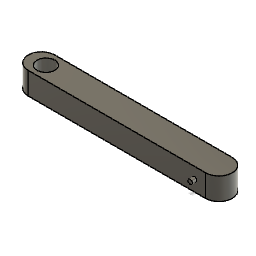
Segunda parte Braço v7 (Autodesk Fusion 360 design; units mm, degrees)
Autodesk Fusion 360 part; units mm, degrees
note: some values were not read from the file. Set by a fixed rule: which sketch regions a step uses.
sketch "Sketch1" plane through (0, 0, 0) normal (0, 1, 0) x (1, 0, 0)
  line L0 (100, -15) -> (-100, -15)
  line L1 (-100, -15) -> (-100, 15)
  line L2 (-100, 15) -> (100, 15)
  line L3 (100, 15) -> (100, -15)
  line L4 (100, -15) -> (-100, 15) construction
  line L5 (-100, -15) -> (100, 15) construction
  arc A0 (-95.599, 14.3399) -> (-95.599, -14.3399) centre (-100, 0) ccw
  arc A1 (95.599, -14.3399) -> (95.599, 14.3399) centre (100, 0) ccw
  dimension "d1" = 200
  dimension "d2" = 30
  constraint horizontal L0
  constraint perpendicular L0 L1
  constraint parallel L0 L2
  constraint parallel L1 L3
  constraint coincident L4 origin
  constraint coincident L5 origin
  constraint midpoint L3 A1.centre
  constraint coincident L2.end A1
  constraint midpoint L1 A0.centre
  constraint coincident L1.end A0
  constraint coincident L5 A0.end
  constraint coincident L4 A0.start
  constraint coincident L5 A1.end
  constraint coincident L4 A1.start
  measures "d1" distance of L1.end L2.end
  measures "d2" distance of L0.end L1.end
extrude "Extrude1" add sketch "Sketch1" along normal blind 25 makes body 1
sketch "Sketch2" plane through (0, 25, 0) normal (0, 1, 0) x (-1, 0, 0)
  arc A0 (100, -15) -> (100, 15) centre (100, 0) ccw
  line L0 (100, 15) -> (-100, 15)
  arc A1 (-100, 15) -> (-100, -15) centre (-100, 0) ccw
  line L1 (-100, -15) -> (100, -15)
  circle A2 centre (95, 0) radius 10
  dimension "d6" = 20
  measures "d6" diameter of A2
extrude "Extrude2" cut sketch "Sketch2" against normal blind 70 contours A2 bodies 1
sketch "Sketch3" plane through (0, 0, -15) normal (0, 0, -1) x (-1, 0, 0)
  line L0 (-100, 0) -> (100, 0)
  line L1 (100, 0) -> (100, 25)
  line L2 (100, 25) -> (-100, 25)
  line L3 (-100, 25) -> (-100, 0)
  line L4 (-85, 15.675) -> (-85, 15.5847)
  line L5 (-86.7208, 15.1734) -> (-85, 15.1734)
  line L6 (-83.2872, 15.1734) -> (-83.2758, 15.1734)
  line L7 (-85, 15.1734) -> (-83.2758, 15.1734)
  arc A0 (-86.7128, 15.1734) -> (-83.2872, 15.1734) centre (-85, 12.5) ccw
  dimension "d11" = 6.35
  dimension "d18" = 3.445
  constraint perpendicular L4 L5
  constraint collinear L5 L6
  constraint parallel L6 L7
  constraint coincident L5 A0.start
  measures "d11" diameter of A0
  measures "d18" distance of L5.start L6.end
extrude "Extrude3" cut sketch "Sketch3" against normal blind 14.986 contours L5 L7 A0 bodies 1
sketch "Sketch4" plane through (0, 0, 15) normal (0, 0, 1) x (1, 0, 0)
  line L0 (-100, 0) -> (100, 0)
  line L1 (100, 0) -> (100, 25)
  line L2 (100, 25) -> (-100, 25)
  line L3 (-100, 25) -> (-100, 0)
  circle A0 centre (87.5, 12.5) radius 2.4995
  dimension "d15" = 4.999
  measures "d15" diameter of A0
extrude "Extrude4" add sketch "Sketch4" along normal blind 5 contours A0 bodies 1
copy_body "Body->Comp1" bodies 1 removing the originals makes body 2 in component "Component"
component "Component" placed x (1, 0, 0) y (0, 1, 0) z (0, 0, 1) at (0, 0, 0)
